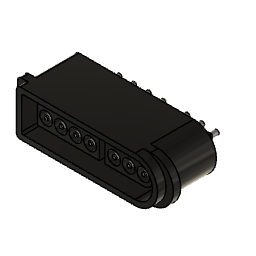
Uzebox Enclosure 2.0 (Autodesk Fusion 360 archive; units mm, degrees)
design "SNES Joypad Connector Type 2"
Autodesk Fusion 360 part; units mm, degrees
sketch "Sketch1" plane through (0, 0, 0) normal (0, 1, 0) x (1, 0, 0)
  line L0 (-17.76, 5.15) -> (-17.76, -5.15)
  line L1 (-16.76, -6.15) -> (14.5, -6.15)
  line L2 (14.5, 6.15) -> (-16.76, 6.15)
  arc A0 (-16.76, 6.15) -> (-17.76, 5.15) centre (-16.76, 5.15) ccw
  arc A1 (-17.76, -5.15) -> (-16.76, -6.15) centre (-16.76, -5.15) ccw
  line L3 (-14.36, -2.75) -> (14.5, -2.75)
  line L4 (14.5, 2.75) -> (-14.36, 2.75)
  circle A2 centre (-12, 0) radius 1.75
  circle A3 centre (14.5, 0) radius 1.75
  circle A4 centre (-8, 0) radius 1.75
  circle A5 centre (-4, 0) radius 1.75
  circle A6 centre (0, 0) radius 1.75
  circle A7 centre (10.5, 0) radius 1.75
  circle A8 centre (6.5, 0) radius 1.75
  circle A9 centre (-12, 0) radius 0.625
  circle A10 centre (-8, 0) radius 0.625
  circle A11 centre (-4, 0) radius 0.625
  circle A12 centre (0, 0) radius 0.625
  circle A13 centre (14.5, 0) radius 0.625
  circle A14 centre (10.5, 0) radius 0.625
  circle A15 centre (6.5, 0) radius 0.625
  line L5 (-15.86, -4.75) -> (14.5, -4.75)
  line L6 (14.5, 4.75) -> (-15.86, 4.75)
  line L7 (-16.36, 4.25) -> (-16.36, -4.25)
  line L8 (-17.76, 0) -> (22.65, 0) construction
  line L9 (-4, 4.75) -> (-4, -4.75) construction
  line L10 (-14.36, -2.75) -> (-14.36, 2.75)
  arc A16 (-15.86, 4.75) -> (-16.36, 4.25) centre (-15.86, 4.25) ccw
  arc A17 (-16.36, -4.25) -> (-15.86, -4.75) centre (-15.86, -4.25) ccw
  line L11 (2.5, 2.75) -> (4, 2.75)
  line L12 (4, 2.75) -> (4, -2.75)
  line L13 (4, -2.75) -> (2.5, -2.75)
  line L14 (2.5, -2.75) -> (2.5, 2.75)
  line L15 (2.5, 2.75) -> (4, -2.75) construction
  line L16 (4, 2.75) -> (2.5, -2.75) construction
  line L17 (14.5, 7.0361) -> (14.5, -7.7499) construction
  arc A18 (14.5, -6.15) -> (14.5, 6.15) centre (14.5, 0) ccw
  arc A19 (14.5, -4.75) -> (14.5, 4.75) centre (14.5, 0) ccw
  arc A20 (14.5, -2.75) -> (14.5, 2.75) centre (14.5, 0) ccw
  arc A21 (16.5, -6.15) -> (16.5, 6.15) centre (16.5, 0) ccw
  line L18 (14.5, 6.15) -> (16.5, 6.15)
  line L19 (14.5, -6.15) -> (16.5, -6.15)
  line L20 (-16.76, 6.15) -> (-18.76, 6.15)
  line L21 (-19.76, 5.15) -> (-19.76, -5.15)
  line L22 (-18.76, -6.15) -> (-16.76, -6.15)
  arc A22 (-18.76, 6.15) -> (-19.76, 5.15) centre (-18.76, 5.15) ccw
  arc A23 (-19.76, -5.15) -> (-18.76, -6.15) centre (-18.76, -5.15) ccw
  point P0 (3.25, 0)
  point P1 (20.65, 0)
  dimension "d6" = 1
  dimension "d31" = 4
  dimension "d32" = 0
  dimension "d35" = -4
  dimension "d36" = 0
  dimension "d45" = 4
  dimension "d46" = 0
  dimension "d50" = -4
  dimension "d51" = 0
  dimension "d89" = 12.3
  dimension "d92" = 1.75
  dimension "d93" = 0.625
  dimension "d94" = 0.625
  dimension "d95" = 1.75
  dimension "d97" = 5.76
  dimension "d98" = 2
  dimension "d99" = 2
  dimension "d100" = 1.4
  dimension "d101" = 2
  dimension "d104" = 0.5
  dimension "d105" = 6.5
  dimension "d106" = 1.5
  dimension "d107" = 3.25
  dimension "d112" = 2
  dimension "d113" = 38.41
  dimension "d114" = 2
  dimension "d116" = 2
  dimension "d117" = 1
  dimension "d118" = 6.15
  dimension "d119" = 12.3
  constraint tangent L0 A0
  constraint tangent L2 A0
  constraint tangent L0 A1
  constraint tangent L1 A1
  constraint equal A0 A1
  constraint horizontal L2
  constraint vertical L0
  constraint horizontal L4
  constraint horizontal L3
  constraint horizontal L8
  constraint concentric A2 A9
  constraint coincident A2.centre L8
  constraint coincident A3.centre L8
  constraint concentric A3 A13
  constraint coincident L6 L9.start
  constraint coincident L5 L9.end
  constraint perpendicular L5 L9
  constraint midpoint A5.centre L9
  constraint vertical L10
  constraint coincident L0 L8.start
  constraint coincident A6.centre A12.centre
  constraint tangent L6 A16
  constraint tangent L7 A16
  constraint tangent L5 A17
  constraint tangent L7 A17
  constraint equal A16 A17
  constraint horizontal L11
  constraint perpendicular L11 L12
  constraint parallel L11 L13
  constraint parallel L12 L14
  constraint coincident L15 P0
  constraint coincident L16 P0
  constraint coincident L8 P0
  constraint collinear L4 L11
  constraint perpendicular L1 L17
  constraint coincident A3.centre L17
  constraint coincident L2.start L17
  constraint coincident L6.start L17
  constraint coincident L4.start L17
  constraint coincident L3.end L17
  constraint coincident L5.end L17
  constraint coincident L1.end L17
  constraint concentric A13 A18
  constraint concentric A13 A19
  constraint concentric A18 A20
  constraint coincident L8 A21.centre
  constraint midpoint A18 P1
  constraint coincident L8.end A21
  constraint tangent A21 L18
  constraint tangent A21 L19
  constraint tangent A0 L20
  constraint perpendicular L20 L21
  constraint perpendicular L21 L22
  constraint tangent L20 A22
  constraint tangent L21 A22
  constraint tangent L21 A23
  constraint tangent L22 A23
  constraint equal A22 A23
  measures "d6" radius of A0
  measures "d89" distance of L1 L2
  measures "d92" radius of A3
  measures "d93" radius of A13
  measures "d94" radius of A9
  measures "d95" radius of A2
  measures "d97" distance of L0 A2.centre
  measures "d98" distance of L4 L6
  measures "d99" distance of L3 L5
  measures "d100" distance of L1 L5
  measures "d101" distance of L7 L10
  measures "d104" radius of A16
  measures "d105" distance of A8.centre A6.centre
  measures "d106" distance of L12.end L13.end
  measures "d107" distance of A6.centre P0
  measures "d112" distance of A3.centre A21.centre
  measures "d113" distance of L0 P1
  measures "d114" distance of L8.end P1
  measures "d116" distance of L0 L21
  measures "d117" radius of A22
  measures "d118" radius of A18
  measures "d119" diameter of A21
extrude "Extrude11" add sketch "Sketch1" along normal blind 2.3 contours L0 L1 L2 A0 A1 A18 makes body 1
extrude "Extrude18" add sketch "Sketch1" along normal blind 2 from surface at 2.3 contours L0 L1 L2 A0 A1 A18 | L0 A0 A1 L20 L21 L22 A22 A23 | A18 A21 L18 L19 | L3 L4 L10 L14 | L3 L4 L12 A20 bodies 1 makes body 2 at (-5.3303, 2.3, 2.415) makes body 3 at (9.6231, 2.3, 2.415)
extrude "Extrude20" add sketch "Sketch1" along normal blind 9.7 from surface at 4.3 contours L0 L1 L2 A0 A1 A18 | L3 L4 L10 L14 | L3 L4 L12 A20 bodies 1 2 3
extrude "Extrude21" add sketch "Sketch1" along normal blind 2 from surface at 14 contours L0 L1 L2 A0 A1 A18 | L3 L4 L10 L14 | L3 L4 L11 L12 L13 L14 | L3 L4 L12 A20 | A2 | A3 | A4 | A5 | A6 | A7 | A8 | L5 L6 L7 A16 A17 A19 bodies 1 2 3
sketch "Sketch6" plane through (0, 16, 0) normal (0, 1, 0) x (-1, 0, 0)
  circle A0 centre (-14.5, 0) radius 0.625
  circle A1 centre (8, 0) radius 0.625
  circle A2 centre (12, 0) radius 0.625
  circle A3 centre (-10.5, 0) radius 0.625
  circle A4 centre (-6.5, 0) radius 0.625
  circle A5 centre (0, 0) radius 0.625
  circle A6 centre (4, 0) radius 0.625
  arc A7 (-14.5, 6.15) -> (-14.5, -6.15) centre (-14.5, 0) ccw
  line L0 (-14.5, -6.15) -> (16.76, -6.15)
  arc A8 (16.76, -6.15) -> (17.76, -5.15) centre (16.76, -5.15) ccw
  line L1 (17.76, -5.15) -> (17.76, 5.15)
  arc A9 (17.76, 5.15) -> (16.76, 6.15) centre (16.76, 5.15) ccw
  line L2 (16.76, 6.15) -> (-14.5, 6.15)
  line L3 (-16.3749, 2.05) -> (14.25, 2.05)
  line L4 (14.25, 2.05) -> (14.25, -2.05)
  line L5 (14.25, -2.05) -> (-16.3749, -2.05)
  line L6 (-16.3749, -2.05) -> (-16.3749, 2.05)
  line L7 (-13.875, -2.05) -> (-15.125, -2.05)
  line L8 (-15.125, -2.05) -> (-15.125, 2.05)
  line L9 (-15.125, 2.05) -> (-13.875, 2.05)
  line L10 (-13.875, 2.05) -> (-13.875, -2.05)
  line L11 (-13.875, -2.05) -> (-15.125, 2.05) construction
  line L12 (-15.125, -2.05) -> (-13.875, 2.05) construction
  line L13 (-9.875, -2.05) -> (-11.125, -2.05)
  line L14 (-11.125, -2.05) -> (-11.125, 2.05)
  line L15 (-11.125, 2.05) -> (-9.875, 2.05)
  line L16 (-9.875, 2.05) -> (-9.875, -2.05)
  line L17 (-9.875, -2.05) -> (-11.125, 2.05) construction
  line L18 (-11.125, -2.05) -> (-9.875, 2.05) construction
  line L19 (-5.875, -2.05) -> (-7.125, -2.05)
  line L20 (-7.125, -2.05) -> (-7.125, 2.05)
  line L21 (-7.125, 2.05) -> (-5.875, 2.05)
  line L22 (-5.875, 2.05) -> (-5.875, -2.05)
  line L23 (-5.875, -2.05) -> (-7.125, 2.05) construction
  line L24 (-7.125, -2.05) -> (-5.875, 2.05) construction
  line L25 (0.625, -2.05) -> (-0.625, -2.05)
  line L26 (-0.625, -2.05) -> (-0.625, 2.05)
  line L27 (-0.625, 2.05) -> (0.625, 2.05)
  line L28 (0.625, 2.05) -> (0.625, -2.05)
  line L29 (0.625, -2.05) -> (-0.625, 2.05) construction
  line L30 (-0.625, -2.05) -> (0.625, 2.05) construction
  line L31 (4.625, -2.05) -> (3.375, -2.05)
  line L32 (3.375, -2.05) -> (3.375, 2.05)
  line L33 (3.375, 2.05) -> (4.625, 2.05)
  line L34 (4.625, 2.05) -> (4.625, -2.05)
  line L35 (4.625, -2.05) -> (3.375, 2.05) construction
  line L36 (3.375, -2.05) -> (4.625, 2.05) construction
  line L37 (8.625, -2.05) -> (7.375, -2.05)
  line L38 (7.375, -2.05) -> (7.375, 2.05)
  line L39 (7.375, 2.05) -> (8.625, 2.05)
  line L40 (8.625, 2.05) -> (8.625, -2.05)
  line L41 (8.625, -2.05) -> (7.375, 2.05) construction
  line L42 (7.375, -2.05) -> (8.625, 2.05) construction
  line L43 (11.375, -2.05) -> (12.625, -2.05)
  line L44 (12.625, -2.05) -> (12.625, 2.05)
  line L45 (12.625, 2.05) -> (11.375, 2.05)
  line L46 (11.375, 2.05) -> (11.375, -2.05)
  line L47 (11.375, -2.05) -> (12.625, 2.05) construction
  line L48 (12.625, -2.05) -> (11.375, 2.05) construction
  point P0 (-14.5, 0)
  point P1 (-10.5, 0)
  point P2 (-6.5, 0)
  point P3 (4, 0)
  point P4 (8, 0)
  point P5 (12, 0)
  dimension "d155" = 4.1
  dimension "d156" = 2.05
  dimension "d157" = 1.8749
  dimension "d158" = 2.25
  constraint horizontal L3
  constraint vertical L4
  constraint horizontal L5
  constraint vertical L6
  constraint horizontal L7
  constraint perpendicular L7 L8
  constraint parallel L7 L9
  constraint parallel L8 L10
  constraint coincident L11 P0
  constraint coincident L12 P0
  constraint coincident L5 L7.start
  constraint coincident P0 A0.centre
  constraint horizontal L13
  constraint perpendicular L13 L14
  constraint parallel L13 L15
  constraint parallel L14 L16
  constraint coincident L17 P1
  constraint coincident L18 P1
  constraint coincident L5 L13.start
  constraint coincident P1 A3.centre
  constraint horizontal L19
  constraint perpendicular L19 L20
  constraint parallel L19 L21
  constraint parallel L20 L22
  constraint coincident L23 P2
  constraint coincident L24 P2
  constraint coincident L5 L19.start
  constraint coincident P2 A4.centre
  constraint horizontal L25
  constraint perpendicular L25 L26
  constraint parallel L25 L27
  constraint parallel L26 L28
  constraint coincident L29 A5.centre
  constraint coincident L30 A5.centre
  constraint coincident L5 L25.start
  constraint coincident A5.centre origin
  constraint horizontal L31
  constraint perpendicular L31 L32
  constraint parallel L31 L33
  constraint parallel L32 L34
  constraint coincident L35 P3
  constraint coincident L36 P3
  constraint coincident L5 L31.start
  constraint coincident P3 A6.centre
  constraint horizontal L37
  constraint perpendicular L37 L38
  constraint parallel L37 L39
  constraint parallel L38 L40
  constraint coincident L41 P4
  constraint coincident L42 P4
  constraint coincident L5 L37.start
  constraint coincident P4 A1.centre
  constraint horizontal L43
  constraint perpendicular L43 L44
  constraint parallel L43 L45
  constraint parallel L44 L46
  constraint coincident L47 P5
  constraint coincident L48 P5
  constraint coincident L5 L43.start
  constraint coincident P5 A2.centre
  constraint tangent A0 L10
  constraint tangent A3 L16
  constraint tangent A4 L22
  constraint tangent A5 L28
  constraint tangent A6 L32
  constraint tangent A1 L38
  constraint tangent A2 L46
  measures "d155" distance of L3 L5
  measures "d156" distance of P5 L3
  measures "d157" distance of P0 L6
  measures "d158" distance of P5 L4
extrude "Extrude22" add sketch "Sketch6" along normal blind 3.1 contours L3 L5 L10 L14 | L3 L5 L6 L8 | L3 L5 L16 L20 | L3 L5 L22 L26 | L3 L5 L28 L32 | L3 L5 L34 L38 | L3 L5 L40 L46 | L3 L4 L5 L44 bodies 1
extrude "Extrude23" add sketch "Sketch6" along normal blind 1.5 contours A0 L5 L7 L8 L10 | A0 L3 L8 L9 L10 | A3 L3 L14 L15 L16 | A3 L5 L13 L14 L16 | A4 L3 L20 L21 L22 | A4 L5 L19 L20 L22 | A5 L3 L26 L27 L28 | A5 L5 L25 L26 L28 | A6 L3 L32 L33 L34 | A6 L5 L31 L32 L34 | A1 L3 L38 L39 L40 | A1 L5 L37 L38 L40 | A2 L3 L44 L45 L46 | A2 L5 L43 L44 L46 bodies 1
extrude "Extrude24" add sketch "Sketch1" along normal blind 20 from surface at 2.3 separate body contours A9 | A10 | A11 | A12 | A13 | A14 | A15 makes body 4 at (7.1242, 15.6333, 0.0312) makes body 5 at (-11.3758, 15.6333, 0.0312) makes body 6 at (0.6242, 15.6333, 0.0312) makes body 7 at (11.1242, 15.6333, 0.0312) makes body 8 at (-7.3758, 15.6333, 0.0312) makes body 9 at (-3.3758, 15.6333, 0.0312) makes body 10 at (15.1242, 15.6333, 0.0312)
fillet "Fillet4" radius 0.2 7 edges at (5.9173, 2.3, 0.226) (-12.5827, 2.3, 0.226) (-0.5827, 2.3, 0.226) (9.9173, 2.3, 0.226) (-8.5827, 2.3, 0.226) (-4.5827, 2.3, 0.226) (13.9173, 2.3, 0.226) on bodies 4 5 6 7 8 9 10
equation "d99 = d98"
equation "d101 = d98"
equation "d107 = d105 / 2"
equation "d156 = d155 / 2"
named bodies: "Connector"
